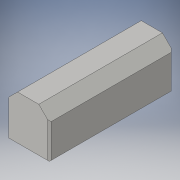
# Autodesk Inventor part: battery_box
Saved by Autodesk Inventor 2016 (Build 200138000, 138)
## iProperties
Created: 2016-02-13
Part Number: battery_box
Material: Generic
Document SubType Name: Modeling
Designer: jforce
Density: 1 g/cm^3
Appearance: Default
Author: jforce
Autodesk Inventor part; units mm, degrees
ref_plane "YZ Plane" through (0, 0, 0) normal (1, 0, 0) x (0, 1, 0)
ref_plane "XZ Plane" through (0, 0, 0) normal (0, 1, 0) x (-1, 0, 0)
ref_plane "XY Plane" through (0, 0, 0) normal (0, 0, 1) x (1, 0, 0)
sketch "Sketch1" plane through (0, 0, 0) normal (0, 0, 1) x (1, 0, 0)
  line L0 (-6, 15) -> (6, 15)
  line L1 (12, 9) -> (12, -10)
  line L2 (10, -12) -> (-10, -12)
  line L3 (-12, -10) -> (-12, 9)
  line L4 (-12, 9) -> (-6, 15)
  line L5 (6, 15) -> (12, 9)
  line L6 (-12, -10) -> (-10, -12)
  line L7 (10, -12) -> (12, -10)
  point P0 (0, 0)
  point P1 (-12, 15)
  point P2 (12, -12)
  point P3 (12, 15)
  point P4 (-12, -12)
  dimension "d0" = 24
  dimension "d1" = 27
  dimension "d2" = 12
  dimension "d3" = 12
  dimension "d4" = 6
  dimension "d5" = 6
  dimension "d6" = 6
  dimension "d7" = 6
  dimension "d8" = 2
  dimension "d9" = 2
  dimension "d10" = 2
  dimension "d11" = 2
  constraints: 16 end point, 8 point on line, 2 parallel, 1 horizontal, 1 perpendicular
  measures "d0" distance of point (-12, 15) point (12, 15)
  measures "d1" distance of point (-12, -12) point (-12, 15)
  measures "d2" distance from line of point (0, 0) L3
  measures "d3" distance from line of point (0, 0) L2
  measures "d4" distance of L3.end point (-12, 15)
  measures "d5" distance of L0.start point (-12, 15)
  measures "d6" distance of L0.end point (12, 15)
  measures "d7" distance of L1.start point (12, 15)
  measures "d8" distance of L3.start point (-12, -12)
  measures "d9" distance of L2.end point (-12, -12)
  measures "d10" distance of L2.start point (12, -12)
  measures "d11" distance of L1.end point (12, -12)
extrude "Extrusion1" add sketch "Sketch1" along normal blind 70
chamfer "Chamfer1" distance 2 angle 45 2 edges at (0, -12, 70) (0, -12, 0)
chamfer "Chamfer2" distance 1 angle 45 4 edges at (12, -0.5, 0) (-12, -0.5, 0) (-12, -0.5, 70) (12, -0.5, 70)
equation "\"d5\" = d4"
equation "\"d6\" = d4"
equation "\"d7\" = d6"
equation "\"d9\" = d8"
equation "\"d10\" = d8"
equation "\"d11\" = d10"
body "Solid1"
